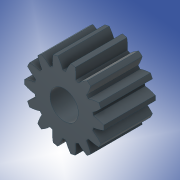
# Autodesk Inventor part: FA010
Saved by Autodesk Inventor 2017 SP1 (Build 210196100, 196)
## iProperties
Created: 2017-06-24
Part Number: FA010
Material: ABS Plastic
Document SubType Name: Modeling
Designer: Zach
Density: 1.06 g/cm^3
Appearance: CR Dark Blue
Author: Zach
Autodesk Inventor part; units mm, degrees
ref_plane "YZ Plane" through (0, 0, 0) normal (1, 0, 0) x (0, 1, 0)
ref_plane "XZ Plane" through (0, 0, 0) normal (0, 1, 0) x (-1, 0, 0)
ref_plane "XY Plane" through (0, 0, 0) normal (0, 0, 1) x (1, 0, 0)
sketch "Sketch1" plane through (0, 0, 0) normal (0, 0, 1) x (1, 0, 0)
  circle A0 centre (0, 0) radius 11.5
  circle A1 centre (0, 0) radius 5.5
  dimension "d0" = 23
  dimension "d1" = 11
  constraints: 2 centre point, 2 coincident
  measures "d0" diameter of A0
  measures "d1" diameter of A1
extrude "Extrusion1" add sketch "Sketch1" along normal blind 20
sketch "Sketch2" plane through (0, 0, 20) normal (0, 0, 1) x (1, 0, 0)
  line L0 (0, 0) -> (25, 0) construction
  circle A0 centre (0, 0) radius 11.5 construction
  arc A1 (15.3248, 0.9) -> (11.3248, 2) centre (9.3856, -12.8741) ccw
  arc A2 (15.3251, -0.9) -> (15.3248, 0.9) centre (-4.6548, -0.0044) ccw
  arc A3 (11.3248, -2) -> (15.3251, -0.9) centre (9.3862, 12.8742) ccw
  arc A4 (11.3248, -2) -> (11.3248, 2) centre (0, 0) ccw
  arc A5 (13.4166, 7.46) -> (9.3355, 6.7156) centre (14.042, -7.5269) ccw
  arc A6 (11.071, 3.1117) -> (9.3355, 6.7156) centre (0, 0) ccw
  arc A7 (11.071, 3.1117) -> (14.198, 5.8385) centre (2.8708, 15.6718) ccw
  arc A8 (14.198, 5.8385) -> (13.4166, 7.46) centre (-4.1919, -2.0236) ccw
  arc A9 (8.8512, 12.5425) -> (5.4972, 10.101) centre (15.9172, -0.6889) ccw
  arc A10 (8.6245, 7.6071) -> (5.4972, 10.101) centre (0, 0) ccw
  arc A11 (8.6245, 7.6071) -> (10.2587, 11.4205) centre (-4.2133, 15.3654) ccw
  arc A12 (10.2587, 11.4205) -> (8.8512, 12.5425) centre (-2.8988, -3.642) ccw
  arc A13 (2.5326, 15.1408) -> (0.5701, 11.4859) centre (14.6398, 6.2855) ccw
  arc A14 (4.4699, 10.5958) -> (0.5701, 11.4859) centre (0, 0) ccw
  arc A15 (4.4699, 10.5958) -> (4.2876, 14.7406) centre (-10.4628, 12.0156) ccw
  arc A16 (4.2876, 14.7406) -> (2.5326, 15.1408) centre (-1.0315, -4.5391) ccw
  arc A17 (-4.2875, 14.7403) -> (-4.4699, 10.5958) centre (10.4629, 12.015) ccw
  arc A18 (-0.5701, 11.4859) -> (-4.4699, 10.5958) centre (0, 0) ccw
  arc A19 (-0.5701, 11.4859) -> (-2.5327, 15.1412) centre (-14.64, 6.2861) ccw
  arc A20 (-2.5327, 15.1412) -> (-4.2875, 14.7403) centre (1.0401, -4.5371) ccw
  arc A21 (-10.2585, 11.4202) -> (-8.6245, 7.6071) centre (4.2136, 15.3648) ccw
  arc A22 (-5.4972, 10.101) -> (-8.6245, 7.6071) centre (0, 0) ccw
  arc A23 (-5.4972, 10.101) -> (-8.8514, 12.5428) centre (-15.9177, -0.6885) ccw
  arc A24 (-8.8514, 12.5428) -> (-10.2585, 11.4202) centre (2.9057, -3.6365) ccw
  arc A25 (-14.1976, 5.8383) -> (-11.071, 3.1117) centre (-2.8703, 15.6714) ccw
  arc A26 (-9.3355, 6.7156) -> (-11.071, 3.1117) centre (0, 0) ccw
  arc A27 (-9.3355, 6.7156) -> (-13.417, 7.4602) centre (-14.0426, -7.5267) ccw
  arc A28 (-13.417, 7.4602) -> (-14.1976, 5.8383) centre (4.1957, -2.0157) ccw
  arc A29 (-15.3248, -0.9) -> (-11.3248, -2) centre (-9.3856, 12.8741) ccw
  arc A30 (-11.3248, 2) -> (-11.3248, -2) centre (0, 0) ccw
  arc A31 (-11.3248, 2) -> (-15.3251, 0.9) centre (-9.3862, -12.8742) ccw
  arc A32 (-15.3251, 0.9) -> (-15.3248, -0.9) centre (4.6548, 0.0044) ccw
  arc A33 (-13.4166, -7.46) -> (-9.3355, -6.7156) centre (-14.042, 7.5269) ccw
  arc A34 (-11.071, -3.1117) -> (-9.3355, -6.7156) centre (0, 0) ccw
  arc A35 (-11.071, -3.1117) -> (-14.198, -5.8385) centre (-2.8708, -15.6718) ccw
  arc A36 (-14.198, -5.8385) -> (-13.4166, -7.46) centre (4.1919, 2.0236) ccw
  arc A37 (-8.8512, -12.5425) -> (-5.4972, -10.101) centre (-15.9172, 0.6889) ccw
  arc A38 (-8.6245, -7.6071) -> (-5.4972, -10.101) centre (0, 0) ccw
  arc A39 (-8.6245, -7.6071) -> (-10.2587, -11.4205) centre (4.2133, -15.3654) ccw
  arc A40 (-10.2587, -11.4205) -> (-8.8512, -12.5425) centre (2.8988, 3.642) ccw
  arc A41 (-2.5326, -15.1408) -> (-0.5701, -11.4859) centre (-14.6398, -6.2855) ccw
  arc A42 (-4.4699, -10.5958) -> (-0.5701, -11.4859) centre (0, 0) ccw
  arc A43 (-4.4699, -10.5958) -> (-4.2876, -14.7406) centre (10.4628, -12.0156) ccw
  arc A44 (-4.2876, -14.7406) -> (-2.5326, -15.1408) centre (1.0315, 4.5391) ccw
  arc A45 (4.2875, -14.7403) -> (4.4699, -10.5958) centre (-10.4629, -12.015) ccw
  arc A46 (0.5701, -11.4859) -> (4.4699, -10.5958) centre (0, 0) ccw
  arc A47 (0.5701, -11.4859) -> (2.5327, -15.1412) centre (14.64, -6.2861) ccw
  arc A48 (2.5327, -15.1412) -> (4.2875, -14.7403) centre (-1.0401, 4.5371) ccw
  arc A49 (10.2585, -11.4202) -> (8.6245, -7.6071) centre (-4.2136, -15.3648) ccw
  arc A50 (5.4972, -10.101) -> (8.6245, -7.6071) centre (0, 0) ccw
  arc A51 (5.4972, -10.101) -> (8.8514, -12.5428) centre (15.9177, 0.6885) ccw
  arc A52 (8.8514, -12.5428) -> (10.2585, -11.4202) centre (-2.9057, 3.6365) ccw
  arc A53 (14.1976, -5.8383) -> (11.071, -3.1117) centre (2.8703, -15.6714) ccw
  arc A54 (9.3355, -6.7156) -> (11.071, -3.1117) centre (0, 0) ccw
  arc A55 (9.3355, -6.7156) -> (13.417, -7.4602) centre (14.0426, 7.5267) ccw
  arc A56 (13.417, -7.4602) -> (14.1976, -5.8383) centre (-4.1957, 2.0157) ccw
  point P0 (15.3452, 0)
  point P1 (13.8256, 6.658)
  point P2 (9.5676, 11.9974)
  point P3 (3.4146, 14.9605)
  point P4 (-3.4146, 14.9605)
  point P5 (-9.5676, 11.9974)
  point P6 (-13.8256, 6.658)
  point P7 (-15.3452, 0)
  point P8 (-13.8256, -6.658)
  point P9 (-9.5676, -11.9974)
  point P10 (-3.4146, -14.9605)
  point P11 (3.4146, -14.9605)
  point P12 (9.5676, -11.9974)
  point P13 (13.8256, -6.658)
  dimension "d4" = 25
  dimension "d5" = 15
  dimension "d6" = 4
  dimension "d7" = 2
  dimension "d8" = 20
  dimension "d9" = 1.8
  dimension "d10" = 15
  dimension "d11" = 2
  dimension "d12" = 4.0004
  dimension "d15" = 360
  constraints: 115 point on circle, 56 centre point, 2 end point, 1 concentric, 1 horizontal, 1 point on line, 183 other
  measures "d4" distance of L0.start L0.end
  measures "d5" radius of A1
  measures "d6" horizontal distance of A1.start A0.start
  measures "d7" distance from line of L0 A0.start
  measures "d8" radius of A2
  measures "d9" distance of A2.start A1.start
  measures "d10" radius of A3
  measures "d11" distance from line of L0 A0.end
  measures "d12" horizontal distance of A0.end A2.start
extrude "Extrusion2" add sketch "Sketch2" against normal blind 20
body "Solid1"
